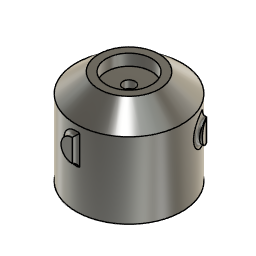
wind_speed_top_center (Autodesk Fusion 360 design; units mm, degrees)
Autodesk Fusion 360 part; units mm, degrees
sketch "Szkic1" plane through (0, 0, 0) normal (0, 1, 0) x (1, 0, 0)
  line L0 (-14, -9.648) -> (-14, 10.352)
  line L1 (-14, -9.648) -> (-10.7329, -7.3965) construction
  line L2 (-14, -9.648) -> (-8, -14.6956)
  line L3 (-10, 10.352) -> (-10, -8.0131)
  line L4 (-10, -8.0131) -> (-8, -9.6956)
  line L5 (-14, 10.352) -> (-10, 10.352)
  line L6 (-10, 7.8472) -> (-14, 10.352) construction
  line L7 (0, -9.6956) -> (-8, -9.6956)
  line L8 (0, -14.6956) -> (-8, -14.6956)
  line L9 (0, -9.6956) -> (0, -14.6956)
  line L10 (0, 0) -> (0, -20.3833)
  line L11 (-4.9, -9.6956) -> (-4.9, -6.6956)
  line L12 (-4.9, -6.6956) -> (-10, -6.6956)
  dimension "d2" = 20
  dimension "d5" = 4
  dimension "d7" = 8
  dimension "d8" = 8
  dimension "d16" = 6
  dimension "d26" = 5
  dimension "d27" = 3
  dimension "d28" = 4.9
  constraint coincident L1 L10.start
  constraint coincident L10.start origin
  constraint perpendicular L3 L5
  constraint parallel L2 L4
  constraint coincident L3 L6.start
  constraint coincident L4 L1.end
  constraint horizontal L7
  constraint coincident L8.start L9.end
  constraint vertical L9
  constraint vertical L10
  constraint collinear L9 L10
  constraint coincident L7 L11.start
  constraint perpendicular L7 L11
  constraint coincident L3 L12.end
  constraint perpendicular L3 L12
  measures "d2" distance of L0.start L0.end
  measures "d5" distance of L0 L3
  measures "d7" distance of L7.start L4.end
  measures "d8" distance of L8.start L2.end
  measures "d16" horizontal distance of L0.start L4.end
  measures "d26" distance of L7 L8
  measures "d27" distance of L11.start L11.end
  measures "d28" horizontal distance of L10.start L11.end
revolve "Obrót1" add sketch "Szkic1" angle 360 about axis through (0, 0, 1.75) along (0, 0, 1)
sketch "Szkic2" plane through (0, 0, 14.6956) normal (0, 0, 1) x (-1, 0, 0)
  circle A0 centre (0, 0) radius 8
  circle A1 centre (0, 0) radius 1.6
  dimension "d9" = 3.2
  constraint coincident A0.centre A1.centre
  measures "d9" diameter of A1
extrude "Wyciągnięcie proste1" cut sketch "Szkic2" against normal blind 5.667 contours A1
sketch "Szkic3" plane through (0, 0, 14.6956) normal (0, 0, 1) x (-1, 0, 0)
  circle A0 centre (0, 0) radius 1.6
  circle A1 centre (0, 0) radius 8
  circle A2 centre (0, 0) radius 6
  dimension "d12" = 12
  constraint coincident A0.centre A1.centre
  measures "d12" diameter of A2
extrude "Wyciągnięcie proste2" cut sketch "Szkic3" against normal blind 3 contours A2
ref_plane "Płaszczyzna konstrukcyjna1" through (0, -14, -0.8921) normal (0, -1, 0) x (1, 0, 0)
sketch "Szkic4" plane through (0, -14, -0.8921) normal (0, -1, 0) x (1, 0, 0)
  line L0 (0, 8) -> (0, 2)
  arc A0 (0, 8) -> (0, 2) centre (0, 5) ccw
  constraint vertical L0
extrude "Wyciągnięcie proste3" add sketch "Szkic4" along normal blind 1 and the other way blind 1
fillet "Zaokrąglenie1" radius 1 2 edges at (-3, -13.6748, 4.1079) (0, -14, 4.1079)
pattern_circular "Szyk kołowy1" count 3 over 360 about axis through (0, 0, 1.75) along (0, 0, 1) of "Wyciągnięcie proste3", "Zaokrąglenie1"
